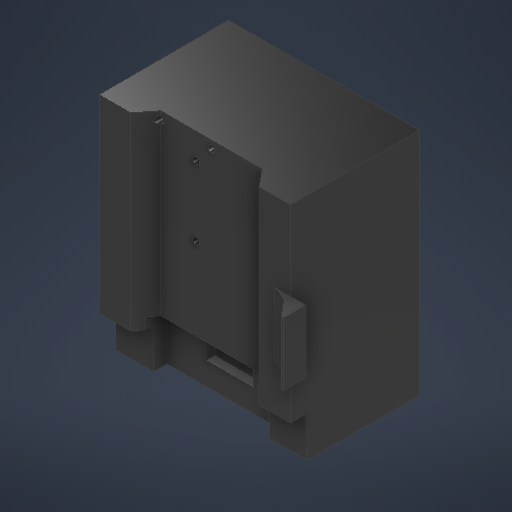
# Autodesk Inventor part: makerbot-shroud
Saved by Autodesk Inventor 2025 (Build 290162000, 162)
## iProperties
Created: 2024-07-16
Part Number: makerbot-shroud
Material: Generic
Document SubType Name: Modeling
Designer: Windows 7 was better
Density: 1 g/cm^3
Appearance: Default
Author: Windows 7 was better
Autodesk Inventor part; units mm, degrees
ref_plane "YZ Plane" through (0, 0, 0) normal (1, 0, 0) x (0, 1, 0)
ref_plane "XZ Plane" through (0, 0, 0) normal (0, 1, 0) x (-1, 0, 0)
ref_plane "XY Plane" through (0, 0, 0) normal (0, 0, 1) x (1, 0, 0)
sketch "Sketch1" plane through (0, 0, 0) normal (0, 0, 1) x (1, 0, 0)
  line L0 (-37.9993, -49.373) -> (47.0007, -49.373)
  line L1 (-37.9993, -49.373) -> (-37.9993, 52.627)
  line L2 (-37.9993, 52.627) -> (47.0007, 52.627)
  line L3 (47.0007, 52.627) -> (47.0007, -49.373)
  line L4 (-37.9993, 52.627) -> (4.5007, 52.627) construction
  line L5 (4.5007, 52.627) -> (4.5007, 50.627) construction
  line L6 (4.5007, 50.627) -> (4.5007, 49.027) construction
  circle A0 centre (4.5007, 49.027) radius 1.6
  line L7 (4.5007, 49.027) -> (27.0007, 49.027) construction
  line L8 (4.5007, 49.027) -> (-17.9993, 49.027) construction
  circle A1 centre (-17.9993, 49.027) radius 1.6
  circle A2 centre (27.0007, 49.027) radius 1.6
  line L9 (-37.9993, 52.627) -> (-2.4993, 52.627) construction
  line L10 (-2.4993, 52.627) -> (-2.4993, 42.627) construction
  line L11 (-2.4993, 42.627) -> (-2.4993, 41.027) construction
  circle A3 centre (-2.4993, 41.027) radius 1.6
  line L12 (-2.4993, 41.027) -> (28.5007, 41.027) construction
  line L13 (-2.4993, 41.027) -> (-2.4993, 10.027) construction
  circle A4 centre (-2.4993, 10.027) radius 1.6
  circle A5 centre (28.5007, 41.027) radius 1.6
  point P0 (0, 0)
  dimension "d0" = 85
  dimension "d1" = 102
  dimension "d2" = 2
  dimension "d3" = 1.6
  dimension "d4" = 3.2
  dimension "d5" = 22.5
  dimension "d6" = 22.5
  dimension "d7" = 3.2
  dimension "d8" = 3.2
  dimension "d9" = 35.5
  dimension "d10" = 10
  dimension "d11" = 1.6
  dimension "d12" = 3.2
  dimension "d13" = 31
  dimension "d14" = 31
  dimension "d15" = 3.2
  dimension "d16" = 3.2
  constraints: 28 end point, 6 centre point, 6 coincident, 4 perpendicular, 4 vertical, 3 horizontal, 1 midpoint, 1 parallel, 1 point on line
  measures "d0" distance of L0.start L0.end
  measures "d1" distance of L0.start L1.end
  measures "d2" distance of L4.end L5.end
  measures "d3" distance of L5.end L6.end
  measures "d4" diameter of A0
  measures "d5" distance of L7.start L7.end
  measures "d6" distance of L7.start L8.end
  measures "d7" diameter of A1
  measures "d8" diameter of A2
  measures "d9" distance of L1.end L9.end
  measures "d10" distance of L9.end L10.end
  measures "d11" distance of L10.end L11.end
  measures "d12" diameter of A3
  measures "d13" distance of L12.start L12.end
  measures "d14" distance of L12.start L13.end
  measures "d15" diameter of A4
  measures "d16" diameter of A5
extrude "Extrusion1" add sketch "Sketch1" along normal blind 50
sketch "Sketch2" plane through (0, 0, 50) normal (0, 0, 1) x (1, 0, 0)
  circle A0 centre (-17.9993, 49.027) radius 1.6 construction
  line L0 (-17.9993, 49.027) -> (-17.9993, 52.627) construction
  line L1 (47.0007, 52.627) -> (-37.9993, 52.627) construction
  circle A1 centre (27.0007, 49.027) radius 1.6 construction
  line L2 (27.0007, 49.027) -> (27.0007, 52.627) construction
  line L3 (-37.9993, -49.4017) -> (-17.9993, -49.4017)
  line L4 (-17.9993, -49.4017) -> (-17.9993, 52.627)
  line L5 (-17.9993, 52.627) -> (-37.9993, 52.627)
  line L6 (-37.9993, 52.627) -> (-37.9993, -49.4017)
  line L7 (47.0007, -49.373) -> (47.0007, 52.627) projected
  line L8 (27.0007, 52.627) -> (47.0007, 52.627)
  line L9 (47.0007, 52.627) -> (47.0007, -49.373)
  line L10 (47.0007, -49.373) -> (27.0007, -49.373)
  line L11 (27.0007, -49.373) -> (27.0007, 52.627)
  point P0 (0, 0)
  constraints: 20 end point, 4 parallel, 2 horizontal, 2 perpendicular, 2 vertical, 1 point on line
extrude "Extrusion2" add sketch "Sketch2" along normal blind 7.5
chamfer "Chamfer1" distance 6 distance2 7.5 1 edges at (-17.9993, 1.6126, 57.5) measured on face at (-18.4993, 1.6126, 57.5)
chamfer "Chamfer2" distance 6 distance2 7.5 1 edges at (27.0007, 1.627, 57.5) measured on face at (27.5007, 1.627, 57.5)
sketch "Sketch3" plane through (0, 0, 0) normal (0, 0, -1) x (-1, 0, 0)
  circle A0 centre (-27.0007, 49.027) radius 1.6 projected
  circle A1 centre (17.9993, 49.027) radius 1.6 projected
  circle A2 centre (-28.5007, 41.027) radius 1.6 projected
  point P0 (0, 0)
extrude "Extrusion3" cut sketch "Sketch3" against normal blind 69.75
sketch "Sketch4" plane through (0, 0, 57.5) normal (0, 0, 1) x (1, 0, 0)
  line L0 (47.0007, 52.627) -> (47.0007, 17.627) construction
  line L1 (47.0007, -49.373) -> (47.0007, 52.627) construction
  line L2 (47.0007, 17.627) -> (54.5007, 17.627)
  line L3 (54.5007, 17.627) -> (54.5007, -10.373)
  line L4 (54.5007, -10.373) -> (47.0007, -10.373)
  line L5 (47.0007, -10.373) -> (47.0007, 17.627)
  line L6 (47.0007, 17.627) -> (40.0007, 17.627)
  line L7 (40.0007, 17.627) -> (40.0007, -10.373)
  line L8 (40.0007, -10.373) -> (47.0007, -10.373)
  line L9 (47.0007, -10.373) -> (47.0007, 17.627)
  point P0 (0, 0)
  dimension "d29" = 35
  dimension "d30" = 7.5
  dimension "d31" = 28
  dimension "d32" = 7
  constraints: 18 end point, 4 parallel, 2 horizontal, 2 perpendicular, 2 point on line
  measures "d29" distance of L0.start L0.end
  measures "d30" distance of L3.end L4.end
  measures "d31" distance of L2.end L3.end
  measures "d32" distance of L8.end L7.end
extrude "Extrusion4" add sketch "Sketch4" along normal blind 3 contours L5 L8 L7 L6
sketch "Sketch5" plane through (0, 0, 57.5) normal (0, 0, 1) x (1, 0, 0)
  line L0 (47.0007, -10.373) -> (47.0007, 17.627) projected
  line L1 (47.0007, 17.627) -> (54.0007, 17.627)
  line L2 (54.0007, 17.627) -> (54.0007, -10.373)
  line L3 (54.0007, -10.373) -> (47.0007, -10.373)
  line L4 (47.0007, -10.373) -> (47.0007, 17.627)
  point P0 (0, 0)
  dimension "d35" = 7
  constraints: 8 end point, 2 parallel, 1 horizontal, 1 perpendicular
  measures "d35" distance of L2.end L3.end
extrude "Extrusion5" add sketch "Sketch5" along normal blind 10
chamfer "Chamfer3" distance 7 distance2 3 1 edges at (40.0007, 3.627, 60.5) measured on face at (40.5007, 3.627, 60.5)
chamfer "Chamfer4" distance 6 distance2 7 1 edges at (47.0007, 3.627, 67.5) measured on face at (47.5007, 3.627, 67.5)
sketch "Sketch6" plane through (0, 0, 50) normal (0, 0, 1) x (1, 0, 0)
  line L0 (47.0007, -49.373) -> (47.0007, -10.373) construction
  line L1 (47.0007, -49.373) -> (17.0007, -49.373) construction
  line L2 (-17.9993, -49.373) -> (27.0007, -49.373) construction
  line L3 (17.0007, -49.373) -> (17.0007, -39.373) construction
  line L4 (17.0007, -39.373) -> (-3.9993, -39.373)
  line L5 (-3.9993, -39.373) -> (-3.9993, -26.373)
  line L6 (-3.9993, -26.373) -> (17.0007, -26.373)
  line L7 (17.0007, -26.373) -> (17.0007, -39.373)
  point P0 (0, 0)
  dimension "d44" = 30
  dimension "d45" = 10
  dimension "d46" = 21
  dimension "d47" = 13
  constraints: 12 end point, 2 parallel, 2 perpendicular, 1 horizontal, 1 point on line
  measures "d44" distance of L0.start L1.end
  measures "d45" distance of L1.end L3.end
  measures "d46" distance of L5.end L6.end
  measures "d47" distance of L4.end L5.end
extrude "Extrusion6" cut sketch "Sketch6" against normal blind 10
sketch "Sketch7" plane through (-37.9993, -49.373, 0) normal (0, -1, 0) x (1, 0, 0)
  line L0 (65, 50) -> (71, 57.5) projected
  line L1 (71, 57.5) -> (85, 57.5) projected
  line L2 (0, 57.5) -> (14, 57.5) projected
  line L3 (14, 57.5) -> (20, 50) projected
  line L4 (0, 50) -> (0, 57.5) projected
  line L5 (0, 50) -> (20, 50) projected
  line L6 (65, 50) -> (85, 50)
  line L7 (85, 50) -> (85, 57.5)
  point P0 (37.9993, 0)
  constraints: 4 end point, 1 horizontal, 1 perpendicular
extrude "Extrusion7" cut sketch "Sketch7" along normal mid plane 36
sketch "Sketch8" plane through (0, 0, 50) normal (0, 0, 1) x (1, 0, 0)
  line L0 (-3.9993, -26.373) -> (17.0007, -26.373) projected
  line L1 (-37.9993, -49.373) -> (47.0007, -49.373) projected
  line L2 (-3.9993, -26.373) -> (30.3139, -26.373)
  line L3 (30.3139, -26.373) -> (30.3139, -49.373)
  line L4 (30.3139, -49.373) -> (-3.9993, -49.373)
  line L5 (-3.9993, -49.373) -> (-3.9993, -26.373)
  line L6 (-3.9993, -26.373) -> (-21.3047, -26.373)
  line L7 (-21.3047, -26.373) -> (-21.3047, -49.373)
  line L8 (-21.3047, -49.373) -> (-3.9993, -49.373)
  line L9 (-3.9993, -49.373) -> (-3.9993, -26.373)
  point P0 (0, 0)
  constraints: 16 end point, 4 parallel, 2 horizontal, 2 perpendicular, 2 point on line
extrude "Extrusion8" cut sketch "Sketch8" along normal mid plane 12
sketch "Sketch10" plane through (0, 0, 50) normal (0, 0, 1) x (1, 0, 0)
  arc A0 (27.0007, 41.5838) -> (27.0007, 40.4702) centre (28.5007, 41.027) ccw projected
  circle A1 centre (28.5007, 41.027) radius 3
  point P0 (0, 0)
  dimension "d57" = 6
  constraints: 1 centre point, 1 coincident
  measures "d57" diameter of A1
extrude "Extrusion10" cut sketch "Sketch10" along normal blind 14
body "Solid1"
